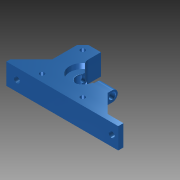
# Autodesk Inventor part: SanladererBowdenBodyMirrored
Saved by Autodesk Inventor 2015 SP1 (Build 190203100, 203)
## iProperties
Created: 2015-01-11
Part Number: SanladererBowdenBodyMirrored
Material: ABS Plastic
Document SubType Name: Modeling
Designer: Jack
Density: 1.06 g/cm^3
Appearance: Cyan
Mass: 23.0198 g
Surface Area: 84.5278 cm^2
Volume: 21.7168 cm^3
Vendor: Jack; Thomas Sanladerer
Author: Jack Cleveland; Thomas Sanladerer
Title: Sanladerer Bowden Extruder Body Mirrored
Autodesk Inventor part; units mm, degrees
ref_plane "YZ Plane" through (0, 0, 0) normal (1, 0, 0) x (0, 1, 0)
ref_plane "XZ Plane" through (0, 0, 0) normal (0, 1, 0) x (-1, 0, 0)
ref_plane "XY Plane" through (0, 0, 0) normal (0, 0, 1) x (1, 0, 0)
sketch "Sketch1" plane through (0, 0, 0) normal (0, 0, 1) x (1, 0, 0)
  line L0 (0, 0) -> (42.2, 0)
  line L1 (0, 0) -> (0, 42.2)
  line L2 (0, 42.2) -> (42.2, 42.2)
  line L3 (42.2, 42.2) -> (42.2, 0)
  dimension "d0" = 42.2
  dimension "d1" = 42.2
  constraints: 8 end point, 2 perpendicular, 1 horizontal, 1 vertical
  measures "d0" distance of L0.start L0.end
  measures "d1" distance of L2.end L0.end
extrude "Extrusion1" add sketch "Sketch1" along normal blind 16
sketch "Sketch2" plane through (0, 0, 16) normal (0, 0, 1) x (1, 0, 0)
  line L0 (0, 0) -> (42.2, 0) projected
  line L1 (42.2, 0) -> (42.2, 42.2) projected
  circle A0 centre (21.1, 21.1) radius 4.8
  dimension "d7" = 9.6
  dimension "d8" = 21.1
  dimension "d9" = 21.1
  constraints: 1 centre point
  measures "d7" diameter of A0
  measures "d8" distance from line of L0 A0.centre
  measures "d9" distance from line of L1 A0.centre
extrude "Extrusion2" cut sketch "Sketch2" against normal up to next
sketch "Sketch3" plane through (0, 0, 16) normal (0, 0, 1) x (1, 0, 0)
  circle A0 centre (21.1, 21.1) radius 4.8 projected
  circle A1 centre (5.6, 36.6) radius 1.75
  circle A2 centre (36.6, 5.6) radius 1.75
  circle A3 centre (5.6, 5.6) radius 1.75
  dimension "d12" = 3.5
  dimension "d14" = 31
  dimension "d15" = 15.5
  dimension "d16" = 15.5
  dimension "d19" = 31
  constraints: 3 centre point, 2 equal radius, 1 horizontal alignment, 1 vertical alignment
  measures "d12" diameter of A1
  measures "d14" distance of A3.centre A1.centre
  measures "d15" horizontal distance of A0.centre A3.centre
  measures "d16" horizontal distance of A3.centre A0.centre
  measures "d19" distance of A2.centre A3.centre
extrude "Extrusion3" cut sketch "Sketch3" against normal up to next contours A1 | A2 | A3
sketch "Sketch4" plane through (0, 0, 16) normal (0, 0, 1) x (1, 0, 0)
  circle A0 centre (21.1, 21.1) radius 4.8 projected
  circle A1 centre (21.1, 21.1) radius 10
  dimension "d20" = 20
  constraints: 1 centre point, 1 coincident
  measures "d20" diameter of A1
extrude "Extrusion4" cut sketch "Sketch4" against normal blind 4
sketch "Sketch5" plane through (0, 0, 16) normal (0, 0, 1) x (1, 0, 0)
  circle A0 centre (21.1, 21.1) radius 10 projected
  circle A1 centre (21.1, 21.1) radius 12.5
  dimension "d23" = 25
  constraints: 1 centre point, 1 coincident
  measures "d23" diameter of A1
extrude "Extrusion5" cut sketch "Sketch5" against normal blind 2
sketch "Sketch6" plane through (0, 0, 16) normal (0, 0, 1) x (1, 0, 0)
  circle A0 centre (21.1, 21.1) radius 12.5 projected
  line L0 (0, 0) -> (42.2, 0) projected
  line L1 (42.2, 0) -> (42.2, 42.2) projected
  line L2 (42.2, 42.2) -> (0, 42.2) projected
  circle A1 centre (21.1, 21.1) radius 4.8 projected
  line L3 (25.4162, 19) -> (42.2, 19)
  line L4 (17.3, 24.0326) -> (17.3, 42.2)
  dimension "d27" = 19
  dimension "d29" = 3.8
  constraints: 4 end point, 2 perpendicular, 2 point on circle, 2 point on line
  measures "d27" distance between parallel lines of L0 L3
  measures "d29" distance from line of A0.centre L4
extrude "Extrusion6" cut sketch "Sketch6" against normal up to next contours A0 L3 A1 L4 | A0 L4 L2 L1 L3 picked at (30.9188, 22.07)
sketch "Sketch7" plane through (0, 0, 12) normal (0, 0, 1) x (1, 0, 0)
  arc A0 (17.3, 30.3499) -> (30.877, 19) centre (21.1, 21.1) ccw projected
  line L0 (42.2, 19) -> (33.4223, 19) projected
  line L1 (39.25, 19) -> (39.25, 29.5)
  line L2 (39.25, 29.5) -> (27.25, 29.5)
  line L3 (27.25, 29.5) -> (27.25, 19)
  line L4 (25.4162, 19) -> (42.2, 19) projected
  point P0 (0, 0)
  dimension "d32" = 6.15
  dimension "d33" = 12
  dimension "d34" = 10.5
  constraints: 6 end point, 2 perpendicular, 2 point on line, 1 vertical
  measures "d32" distance from line of A0.centre L3
  measures "d33" distance of L1.end L2.end
  measures "d34" distance of L1.start L1.end
extrude "Extrusion7" add sketch "Sketch7" against normal blind 8
sketch "Sketch8" plane through (0, 0, 0) normal (0, 0, -1) x (-1, 0, 0)
  arc A0 (-25.4162, 19) -> (-17.3, 24.0326) centre (-21.1, 21.1) ccw projected
  circle A1 centre (-21.1, 21.1) radius 10
  dimension "d37" = 20
  constraints: 1 centre point, 1 coincident
  measures "d37" diameter of A1
extrude "Extrusion8" cut sketch "Sketch8" against normal blind 4
fillet "Fillet1" radius 4 2 edges at (33.25, 29.5, 12) (33.25, 29.5, 4)
chamfer "Chamfer1" distance 4.5 angle 45 1 edges at (0, 42.2, 8)
sketch "Sketch9" plane through (39.25, 19, 12) normal (1, 0, 0) x (0, 0, -1)
  arc A0 (8, 6.5) -> (0, 6.5) centre (4, 6.5) ccw projected
  circle A1 centre (4, 6.5) radius 2.4
  point P0 (12, -19)
  dimension "d45" = 4.8
  constraints: 1 centre point, 1 coincident
  measures "d45" diameter of A1
extrude "Extrusion9" cut sketch "Sketch9" against normal blind 10
sketch "Sketch10" plane through (29.25, 25.5, 8) normal (1, 0, 0) x (0, 0, -1)
  circle A0 centre (0, 0) radius 2.4 projected
  circle A1 centre (0, 0) radius 1.25
  point P0 (8, -25.5)
  dimension "d48" = 2.5
  constraints: 1 centre point, 1 coincident
  measures "d48" diameter of A1
extrude "Extrusion10" cut sketch "Sketch10" against normal up to surface (2 mm away) contours A1
sketch "Sketch11" plane through (17.3, 24.0326, 12) normal (1, 0, 0) x (0, 0, -1)
  circle A0 centre (4, 1.4674) radius 1.25 projected
  circle A1 centre (4, 1.4674) radius 2
  point P0 (12, -24.0326)
  dimension "d51" = 4
  constraints: 1 centre point, 1 coincident
  measures "d51" diameter of A1
extrude "Extrusion11" cut sketch "Sketch11" against normal up to surface (17.3 mm away) contours A0 | A1
sketch "Sketch12" plane through (0, 0, 0) normal (-1, 0, 0) x (0, 0, 1)
  circle A0 centre (8, 25.5) radius 2 projected
  circle A1 centre (8, 25.5) radius 6.25
  dimension "d54" = 12.5
  constraints: 1 centre point, 1 coincident
  measures "d54" diameter of A1
extrude "Extrusion12" cut sketch "Sketch12" against normal blind 7
chamfer "Chamfer2" distance 1 angle 45 1 edges at (0, 25.5, 1.75)
fillet "Fillet3" radius 2.5 1 edges at (7, 25.5, 10)
chamfer "Chamfer3" distance 0.5 angle 45 1 edges at (27.25, 25.5, 9.25)
chamfer "Chamfer4" distance 1 angle 45 3 edges at (35.0635, 19, 12) (39.25, 19, 8) (35.0635, 19, 4)
fillet "Fillet4" radius 0.5 1 edges at (39.25, 25.5, 10.4)
fillet "Fillet5" radius 3.4 1 edges at (25.4162, 19, 8)
fillet "Fillet6" radius 4 1 edges at (27.25, 19, 8)
fillet "Fillet7" radius 0.5 11 edges at (24.9971, 18.2051, 12) (18.0216, 17.4171, 12) (27.25, 23.6845, 12) (27.25, 28.3285, 10.8285) (27.25, 29.5, 8) (27.25, 28.3285, 5.1715) (27.25, 23.6845, 4) (26.7501, 19.9327, 4) (24.9971, 18.2051, 4) (18.0216, 17.4171, 4) (26.7501, 19.9327, 12)
sketch "Sketch13" plane through (0, 0, 16) normal (0, 0, 1) x (1, 0, 0)
  line L0 (0, 37.7) -> (0, 0) projected
  line L1 (42.2, 0) -> (42.2, 19) projected
  line L2 (42.2, 19) -> (61.2, 0)
  line L3 (61.2, 0) -> (42.2, 0)
  line L4 (0, 19) -> (-19, 0)
  line L5 (-19, 0) -> (0, 0)
  dimension "d71" = 45
  dimension "d72" = 45
  constraints: 8 end point, 2 horizontal, 1 horizontal alignment, 1 point on line
  measures "d71" angle of L2 L1
  measures "d72" angle of L0 L4
extrude "Extrusion13" add sketch "Sketch13" against normal up to surface (16 mm away)
sketch "Sketch14" plane through (0, 37.7, 0) normal (-1, 0, 0) x (0, 0, 1)
  circle A0 centre (8, -12.2) radius 7.25 projected
  circle A1 centre (8, -12.2) radius 1.75 projected
  circle A2 centre (8, -12.2) radius 9
  point P0 (0, -37.7)
  dimension "d75" = 18
  constraints: 1 centre point, 1 coincident
  measures "d75" diameter of A2
extrude "Extrusion14" cut sketch "Sketch14" along normal blind 3.5 contours A0 | A2
ref_plane "Work Plane3" through (54.5, 0, 8) normal (-0.809017, -0.5877853, 0) x (0, 0, -1)
sketch "Sketch15" plane through (54.5, 0, 8) normal (-0.809017, -0.5877853, 0) x (0, 0, -1)
  circle A0 centre (0, -8.0618) radius 5.5
  line L0 (-8, -43.2022) -> (-8, 3.9382) projected
  line L1 (-8, 3.9382) -> (8, 3.9382) projected
  point P0 (8, -32.0343)
  dimension "d81" = 11
  dimension "d82" = 8
  dimension "d83" = 12
  constraints: 1 centre point
  measures "d81" diameter of A0
  measures "d82" distance from line of L0 A0.centre
  measures "d83" distance from line of L1 A0.centre
extrude "Extrusion15" cut sketch "Sketch15" against normal blind 4.5
chamfer "Chamfer5" distance 0.5 angle 45 1 edges at (52.6089, 8.5911, 13.5)
sketch "Sketch16" plane through (0, 0, 16) normal (0, 0, 1) x (1, 0, 0)
  line L0 (-19, 0) -> (61.2, 0) projected
  line L1 (-16, 0) -> (-16, 3)
  line L2 (-19, 0) -> (0, 19) projected
  point P0 (0, 0)
  dimension "d89" = 3
  constraints: 2 end point, 2 point on line, 1 vertical
  measures "d89" distance of L1.start L1.end
extrude "Extrusion16" cut sketch "Sketch16" against normal up to next
sketch "Sketch17" plane through (0, 0, 16) normal (0, 0, 1) x (1, 0, 0)
  line L0 (-16, 0) -> (61.2, 0) projected
  line L1 (61.2, 0) -> (42.2, 19) projected
  line L2 (57.2, 4) -> (57.2, 0)
  point P0 (0, 0)
  dimension "d92" = 4
  constraints: 2 end point, 2 point on line, 1 perpendicular
  measures "d92" distance of L2.start L2.end
extrude "Extrusion17" cut sketch "Sketch17" against normal up to next
ref_plane "Work Plane4" through (-16, 5, 0) normal (0, -1, 0) x (1, 0, 0)
sketch "Sketch20" plane through (-16, 0, 0) normal (0, -1, 0) x (1, 0, 0)
  line L0 (0, 16) -> (73.2, 16) projected
  line L1 (0, 16) -> (0, 0) projected
  circle A0 centre (8, 8) radius 2.25
  point P0 (16, 0)
  dimension "d103" = 4.5
  dimension "d104" = 8
  dimension "d105" = 8
  constraints: 1 centre point
  measures "d103" diameter of A0
  measures "d104" distance from line of L0 A0.centre
  measures "d105" distance from line of L1 A0.centre
extrude "Extrusion19" cut sketch "Sketch20" against normal blind 13.5
ref_plane "Work Plane5" through (-16, 4, 0) normal (0, -1, 0) x (1, 0, 0)
sketch "Sketch21" plane through (-16, 4, 0) normal (0, -1, 0) x (1, 0, 0)
  circle A0 centre (8, 8) radius 2.25 projected
  circle A1 centre (8, 8) radius 5
  point P0 (16, 0)
  dimension "d109" = 10
  constraints: 1 centre point, 1 coincident
  measures "d109" diameter of A1
extrude "Extrusion20" cut sketch "Sketch21" against normal blind 12
sketch "Sketch22" plane through (57.2, 0, 16) normal (1, 0, 0) x (0, 0, -1)
  line L0 (16, 4) -> (16, 0) projected
  line L1 (0, 4) -> (16, 4) projected
  line L2 (0, 0) -> (0, 4) projected
  line L3 (16, 0) -> (0, 0) projected
extrude "Extrusion21" add sketch "Sketch22" along normal blind 12
sketch "Sketch23" plane through (57.2, 4, 16) normal (0, 1, 0) x (1, 0, 0)
  line L0 (12, 16) -> (12, 0) projected
  line L1 (0, 16) -> (12, 16) projected
  circle A0 centre (7, 8) radius 2.25
  point P0 (-57.2, 16)
  dimension "d114" = 4.5
  dimension "d115" = 5
  dimension "d116" = 8
  constraints: 1 centre point
  measures "d114" diameter of A0
  measures "d115" distance from line of L0 A0.centre
  measures "d116" distance from line of L1 A0.centre
extrude "Extrusion22" cut sketch "Sketch23" against normal up to next
sketch "Sketch24" plane through (0, 0, 16) normal (0, 0, 1) x (1, 0, 0)
  line L0 (17.3, 33.0084) -> (17.3, 42.2) projected
  line L1 (17.3, 42.2) -> (4.5, 42.2) projected
  line L2 (0, 37.7) -> (0, 19) projected
  line L3 (33.4223, 19) -> (30.877, 19) projected
  arc A0 (17.3, 30.3499) -> (30.877, 19) centre (21.1, 21.1) ccw projected
  line L4 (17.3, 30.3499) -> (17.3, 33.0084) projected
  arc A1 (17.3, 33.0084) -> (33.4223, 19) centre (21.1, 21.1) ccw projected
  line L5 (27.75, 21.869) -> (27.75, 25.5) projected
  arc A2 (25.641, 18.0568) -> (27.75, 21.869) centre (23.25, 21.869) ccw projected
  arc A3 (25.641, 18.0568) -> (25.031, 17.5451) centre (27.1819, 15.6) ccw projected
  arc A4 (17.3, 24.7946) -> (25.031, 17.5451) centre (21.1, 21.1) ccw projected
  line L6 (17.3, 24.7946) -> (17.3, 30.3499) projected
  arc A5 (17.3, 30.3499) -> (31.0393, 20) centre (21.1, 21.1) ccw projected
  line L7 (39.25, 20) -> (31.0393, 20) projected
  line L8 (39.25, 20) -> (39.25, 25.5) projected
  line L9 (27.75, 25.5) -> (39.25, 25.5) projected
  line L10 (13.85, 42.2) -> (13.85, 26.7)
  arc A6 (17.3, 24.7946) -> (25.031, 17.5451) centre (21.1, 21.1) ccw projected
  line L11 (13.85, 26.7) -> (17.3, 26.7)
  arc A7 (13.85, 32.9022) -> (17.3, 26.7) centre (21.15, 32.9022) ccw
  line L12 (17.3, 26.7) -> (17.3, 42.2)
  line L13 (17.3, 42.2) -> (13.85, 42.2)
  point P0 (0, 0)
  dimension "d119" = 13.85
  dimension "d120" = 15.5
  dimension "d121" = 7.3
  constraints: 8 end point, 3 point on line, 2 collinear, 2 point on circle, 1 centre point, 1 horizontal, 1 tangent, 1 vertical
  measures "d119" distance between parallel lines of L2 L10
  measures "d120" distance between parallel lines of L1 L11
  measures "d121" radius of A7
extrude "Extrusion23" cut sketch "Sketch24" against normal up to next contours A1 A7 L10 L1 L0 | L4 A0 A7 A1 | L6 A7 A0
mirror "Mirror1" about plane through (21.1, 21.1, 16) normal (0, 0, 1) remove original yes
ref_plane "Work Plane1" through (42.2, 19, 8) normal (1, 0, 0) x (0, 0, 1)
ref_plane "Work Plane2" through (54.5, 19, 8) normal (1, 0, 0) x (0, 0, 1)
body "Solid1"
